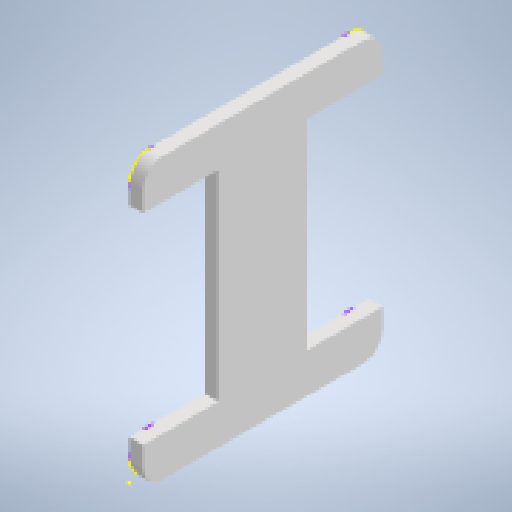
# Autodesk Inventor part: base
Saved by Autodesk Inventor 2025.2 (Build 292293000, 293)
## iProperties
Created: 2025-02-22
Part Number: base
Material: Générique
Document SubType Name: Modeling
Designer: antoi
Density: 1 g/cm^3
Appearance: Par défaut
Author: antoi
Autodesk Inventor part; units mm, degrees
ref_plane "YZ Plane" through (0, 0, 0) normal (1, 0, 0) x (0, 1, 0)
ref_plane "XZ Plane" through (0, 0, 0) normal (0, 1, 0) x (-1, 0, 0)
ref_plane "XY Plane" through (0, 0, 0) normal (0, 0, 1) x (1, 0, 0)
sketch "Esquisse1" plane through (0, 0, 0) normal (1, 0, 0) x (0, 1, 0)
  line L0 (10, 0) -> (131.4, 0)
  line L1 (141.4, -10) -> (141.4, -111)
  line L2 (131.4, -121) -> (10, -121)
  line L3 (0, -111) -> (0, -10)
  arc A0 (131.4, -121) -> (141.4, -111) centre (131.4, -111) ccw
  arc A1 (0, -111) -> (10, -121) centre (10, -111) ccw
  arc A2 (10, 0) -> (0, -10) centre (10, -10) ccw
  arc A3 (141.4, -10) -> (131.4, 0) centre (131.4, -10) ccw
  line L4 (20, -38) -> (121.4, -38)
  line L5 (121.4, -38) -> (121.4, -83)
  line L6 (121.4, -83) -> (20, -83)
  line L7 (20, -83) -> (20, -38)
  circle A4 centre (10, -111) radius 10
  circle A5 centre (131.4, -111) radius 10
  circle A6 centre (131.4, -10) radius 10
  circle A7 centre (10, -10) radius 10
  line L8 (20, -38) -> (20, 0)
  line L9 (20, -83) -> (20, -121)
  line L10 (121.4, -83) -> (121.4, -121)
  line L11 (121.4, -38) -> (121.4, 0)
  point P0 (0, 0)
  point P1 (141.4, -121)
  point P2 (141.4, 0)
  point P3 (0, -121)
  point P4 (70.7, -83)
  dimension "d0" = 141.4
  dimension "d1" = 121
  dimension "d2" = 10
  dimension "d3" = 10
  dimension "d4" = 101.4
  dimension "d5" = 45
  dimension "d11" = 38
  dimension "d12" = 38
  dimension "d13" = 20
  constraints: 24 end point, 14 point on line, 8 centre point, 8 point on circle, 8 tangent, 4 coincident, 4 parallel, 4 perpendicular, 3 equal radius, 2 horizontal, 1 midpoint
  measures "d0" distance of point (141.4, -121) point (0, -121)
  measures "d1" distance of point (141.4, 0) point (141.4, -121)
  measures "d2" radius of A0
  measures "d3" radius of A1
  measures "d4" distance of L5.end L6.end
  measures "d5" distance of L4.end L5.end
  measures "d11" distance between parallel lines of L0 L4
  measures "d12" distance from line of L2 point (70.7, -83)
  measures "d13" distance between parallel lines of L1 L10
extrude "Extrusion1" add sketch "Esquisse1" along normal blind 7 contours A7 A2 | L0 L8 A7 | A7 L8 L7 L9 A4 L3 | L0 A6 L11 | A4 A1 | L4 L5 L6 L7 | A3 A6 | A6 L1 A5 L10 L5 L11 | A4 L9 L2 | A0 A5 | L10 A5 L2
sketch "Esquisse2" plane through (0, 0, 0) normal (-1, 0, 0) x (0, 0, 1)
  line L0 (-42.21, 24.98) -> (-78.79, 24.98)
  line L1 (-78.79, 24.98) -> (-78.79, 68.16)
  line L2 (-78.79, 68.16) -> (-42.21, 68.16)
  line L3 (-42.21, 68.16) -> (-42.21, 24.98)
  line L4 (-42.21, 73.24) -> (-78.79, 73.24)
  line L5 (-78.79, 73.24) -> (-78.79, 116.42)
  line L6 (-78.79, 116.42) -> (-42.21, 116.42)
  line L7 (-42.21, 116.42) -> (-42.21, 73.24)
  line L8 (-38, 121.4) -> (-38, 20) projected
  line L9 (-83, 20) -> (-83, 121.4) projected
  circle A0 centre (-78.79, 24.98) radius 2.3
  circle A1 centre (-42.21, 24.98) radius 2.3
  circle A2 centre (-42.21, 68.16) radius 2.3
  circle A3 centre (-78.79, 68.16) radius 2.3
  circle A4 centre (-78.79, 73.24) radius 2.3
  circle A5 centre (-42.21, 73.24) radius 2.3
  circle A6 centre (-42.21, 116.42) radius 2.3
  circle A7 centre (-78.79, 116.42) radius 2.3
  point P0 (0, 0)
  point P1 (-78.79, 46.57)
  dimension "d8" = 36.58
  dimension "d9" = 43.18
  dimension "d10" = 43.18
  dimension "d14" = 4.21
  dimension "d15" = 4.21
  dimension "d16" = 5.08
  dimension "d17" = 4.6
  dimension "d18" = 4.6
  dimension "d19" = 4.6
  dimension "d20" = 4.6
  dimension "d21" = 4.6
  dimension "d22" = 4.6
  dimension "d23" = 4.6
  dimension "d24" = 4.6
  constraints: 16 end point, 8 centre point, 8 coincident, 4 parallel, 2 horizontal, 2 perpendicular, 1 midpoint, 1 point on line
  measures "d8" distance of L1.end L2.end
  measures "d9" distance of L0.end L1.end
  measures "d10" distance of L4.end L5.end
  measures "d14" distance between parallel lines of L8 L3
  measures "d15" distance from line of L9 point (-78.79, 46.57)
  measures "d16" distance between parallel lines of L2 L4
  measures "d17" diameter of A0
  measures "d18" diameter of A1
  measures "d19" diameter of A2
  measures "d20" diameter of A3
  measures "d21" diameter of A4
  measures "d22" diameter of A5
  measures "d23" diameter of A6
  measures "d24" diameter of A7
extrude "Extrusion2" cut sketch "Esquisse2" against normal blind 5.7 contours A0 L1 L0 | L0 L1 A0 | A1 L3 L0 | L0 L3 A1 | A3 L2 L1 | L1 L2 A3 | A2 L2 L3 | L3 L2 A2 | A4 L5 L4 | L4 L5 A4 | A5 L7 L4 | L4 L7 A5 | A7 L6 L5 | L5 L6 A7 | A6 L6 L7 | L7 L6 A6
sketch "Esquisse3" plane through (0, 0, 0) normal (-1, 0, 0) x (0, 0, 1)
  arc A0 (-10, 0) -> (0, 10) centre (-10, 10) ccw projected
  circle A1 centre (-10, 10) radius 10
  arc A2 (-121, 10) -> (-111, 0) centre (-111, 10) ccw projected
  circle A3 centre (-111, 10) radius 10
  arc A4 (-111, 141.4) -> (-121, 131.4) centre (-111, 131.4) ccw projected
  circle A5 centre (-111, 131.4) radius 10
  arc A6 (0, 131.4) -> (-10, 141.4) centre (-10, 131.4) ccw projected
  circle A7 centre (-10, 131.4) radius 10
  point P0 (0, 0)
  point P1 (-10, 0)
  point P2 (-121, 131.4)
  point P3 (-111, 141.4)
  constraints: 4 centre point, 4 coincident
extrude "Extrusion3" add sketch "Esquisse3" along normal blind 10
fillet "Congé1" radius 10 4 edges at (3.5, 121.4, 0) (3.5, 20, 0) (3.5, 121.4, -121) (3.5, 20, -121)
hole "Perçage1" at (-10, 10, -111) direction (1, 0, 0) diameter 6.3 depth 10
hole "Perçage2" at (-10, 10, -10) direction (1, 0, 0) diameter 6.3 depth 10
hole "Perçage3" at (-10, 131.4, -10) direction (1, 0, 0) diameter 6.3 depth 10
hole "Perçage4" at (-10, 131.4, -111) direction (1, 0, 0) diameter 6.3 depth 10
